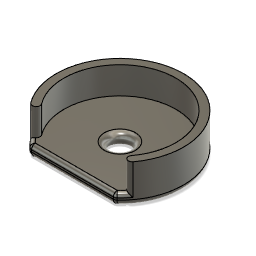
Motor cover v2 (Autodesk Fusion 360 design; units mm, degrees)
Autodesk Fusion 360 part; units mm, degrees
sketch "Sketch1" plane through (0, 0, 0) normal (0, 1, 0) x (1, 0, 0)
  line L0 (-11, -12.298374) -> (11, -12.298374)
  arc A0 (11, -12.298374) -> (-11, -12.298374) centre (0, 0) ccw
  dimension "d1" = 33
  constraint coincident A0.centre origin
  measures "d1" diameter of A0
extrude "Extrude1" add sketch "Sketch1" along normal blind 3 contours L0 A0 picked at (5.206219, -5.269858)
sketch "Sketch2" plane through (0, 3, 0) normal (0, 1, 0) x (-1, 0, 0)
  arc A0 (-11, 12.298374) -> (11, 12.298374) centre (0, 0) ccw
  line L0 (11, 12.298374) -> (-11, 12.298374)
  arc A1 (-10.255312, 10.250784) -> (10.207522, 10.298374) centre (0, 0) ccw
  arc A2 (-12.929479, 10.250784) -> (12.891606, 10.298374) centre (0, 0) ccw
  line L1 (10.207522, 10.298374) -> (12.891606, 10.298374)
  line L2 (-10.255312, 10.250784) -> (-12.929479, 10.250784)
  constraint concentric A0 A1
  constraint horizontal L1
  constraint parallel L0 L2
extrude "Extrude2" add sketch "Sketch2" along normal blind 7 contours A0 A1 A2 L1 L2 picked at (-12.963783, 9.031511)
sketch "Sketch3" plane through (0, 3, 0) normal (0, 1, 0) x (-1, 0, 0)
  line L0 (-12.929479, 10.250784) -> (-10.255312, 10.250784)
  arc A0 (-10.255312, 10.250784) -> (10.207522, 10.298374) centre (0, 0) ccw
  line L1 (10.207522, 10.298374) -> (12.891606, 10.298374)
  arc A1 (12.891606, 10.298374) -> (11, 12.298374) centre (0, 0) ccw
  line L2 (11, 12.298374) -> (-11, 12.298374)
  arc A2 (-11, 12.298374) -> (-12.929479, 10.250784) centre (0, 0) ccw
  circle A3 centre (0, 0) radius 2.5
  dimension "d21" = 5
  constraint coincident A0.centre A1.centre
  measures "d21" diameter of A3
extrude "Extrude4" cut sketch "Sketch3" against normal blind 10 contours A3 picked at (-0.886301, 0.232065)
fillet "Fillet1" radius 1 2 edges at (-10.207522, 6.5, 10.298374) (10.255312, 6.5, 10.250784)
fillet "Fillet2" radius 1.5 2 edges at (0, 0, -16.5) (0, 0, 12.298374)
fillet "Fillet5" radius 1 3 edges at (-11.987586, 3, 11.337892) (0, 3, 12.298374) (12.008462, 3, 11.315779)
fillet "Fillet6" radius 1 2 edges at (-12.891606, 6, 10.298374) (12.929479, 6, 10.250784)
fillet "Fillet7" radius 1.5 2 edges at (2.330818, 0, -0.904039) (2.330818, 3, 0.904039)
fillet "Fillet8" radius 1 6 edges at (-10.823834, 0.421466, 11.840858) (-11, 1.75, 12.298374) (-10.883014, 2.718669, 11.993728) (10.823834, 0.421466, 11.840858) (11, 1.75, 12.298374) (10.883014, 2.718669, 11.993728)
